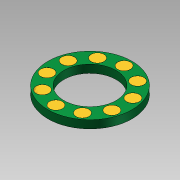
# Autodesk Inventor part: Capsule.contactring
Saved by Autodesk Inventor 2011 (Build 150239000, 239)
## iProperties
Created: 2011-03-22
Part Number: Capsule.contactring
Document SubType Name: Modeling
Designer: Casey
Density: 1 g/cm^3
Author: Casey
Autodesk Inventor part; units mm, degrees
ref_plane "YZ Plane" through (0, 0, 0) normal (1, 0, 0) x (0, 1, 0)
ref_plane "XZ Plane" through (0, 0, 0) normal (0, 1, 0) x (-1, 0, 0)
ref_plane "XY Plane" through (0, 0, 0) normal (0, 0, 1) x (1, 0, 0)
sketch "Sketch1" plane through (0, 0, 0) normal (0, 0, 1) x (1, 0, 0)
  circle A0 centre (0, 0) radius 9.25
  circle A1 centre (0, 0) radius 5.75
  dimension "d0" = 11.5
  dimension "d1" = 18.5
  constraints: 2 centre point, 2 coincident
  measures "d0" diameter of A1
  measures "d1" diameter of A0
extrude "Extrusion1" add sketch "Sketch1" along normal blind 1.75
sketch "Sketch2" plane through (0, 0, 1.75) normal (0, 0, 1) x (1, 0, 0)
  circle A0 centre (0, 0) radius 5.75 projected
  circle A1 centre (0, 7.5) radius 1.4
  dimension "d4" = 7.5
  dimension "d5" = 2.8
  constraints: 1 centre point
  measures "d4" distance of A0.centre A1.centre
  measures "d5" diameter of A1
extrude "Extrusion2" add sketch "Sketch2" along normal blind 0.01 contours A1
pattern_circular "Circular Pattern1" count 10 over 360 about axis through (0, 0, 0) along (0, 0, 1) of "Extrusion2"
body "Solid1"
